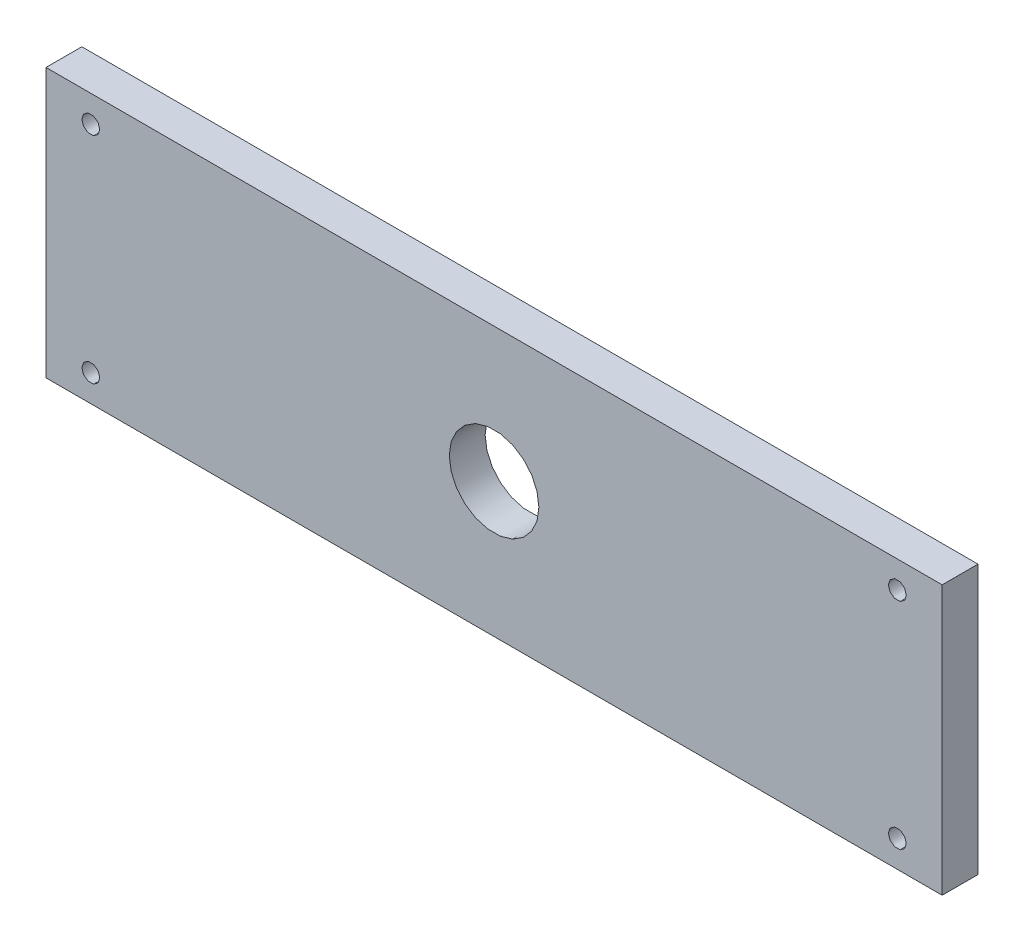
# Autodesk Inventor part: HA03
Saved by Autodesk Inventor 2017 (Build 210142000, 142)
## iProperties
Created: 2018-10-22
Part Number: HA03
Material: ABS Plastic
Document SubType Name: Modeling
Designer: Dell
Density: 1.06 g/cm^3
Appearance: Smooth - Black
Author: Dell
Autodesk Inventor part; units mm, degrees
ref_plane "YZ Plane" through (0, 0, 0) normal (1, 0, 0) x (0, 1, 0)
ref_plane "XZ Plane" through (0, 0, 0) normal (0, 1, 0) x (-1, 0, 0)
ref_plane "XY Plane" through (0, 0, 0) normal (0, 0, 1) x (1, 0, 0)
sketch "Sketch1" plane through (0, 0, 0) normal (0, 0, 1) x (1, 0, 0)
  line L0 (0, 0) -> (250, 0)
  line L1 (250, 0) -> (250, 75)
  line L2 (250, 75) -> (0, 75)
  line L3 (0, 75) -> (0, 0)
  line L4 (12.5, 67.5) -> (237.5, 67.5) construction
  line L5 (237.5, 67.5) -> (237.5, 7.5) construction
  line L6 (237.5, 7.5) -> (12.5, 7.5) construction
  line L7 (12.5, 7.5) -> (12.5, 67.5) construction
  circle A0 centre (12.5, 67.5) radius 2.5
  circle A1 centre (12.5, 7.5) radius 2.5
  circle A2 centre (237.5, 7.5) radius 2.5
  circle A3 centre (237.5, 67.5) radius 2.5
  circle A4 centre (125, 37.5) radius 12.5
  point P0 (125, 67.5)
  point P1 (125, 75)
  point P2 (12.5, 37.5)
  point P3 (0, 37.5)
  dimension "d0" = 250
  dimension "d1" = 75
  dimension "d2" = 225
  dimension "d3" = 60
  dimension "d4" = 5
  dimension "d5" = 5
  dimension "d6" = 5
  dimension "d7" = 5
  dimension "d8" = 25
  constraints: 16 end point, 5 centre point, 4 coincident, 4 midpoint, 4 parallel, 2 horizontal, 2 horizontal alignment, 2 perpendicular, 2 vertical alignment
  measures "d0" distance of L2.end L1.end
  measures "d1" distance of L1.end L0.end
  measures "d2" distance of L4.start L4.end
  measures "d3" distance of L6.end L4.start
  measures "d4" diameter of A0
  measures "d5" diameter of A1
  measures "d6" diameter of A2
  measures "d7" diameter of A3
  measures "d8" diameter of A4
extrude "Extrusion1" add sketch "Sketch1" along normal blind 10
body "Solid1"
